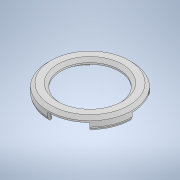
# Autodesk Inventor part: mirror_lock_v3
Saved by Autodesk Inventor 2020 (Build 240168000, 168)
## iProperties
Created: 2024-03-24
Part Number: mirror_lock_v3
Material: Типовые
Document SubType Name: Modeling
Designer: 4s
Density: 1 g/cm^3
Appearance: По умолчанию
Author: 4s
Autodesk Inventor part; units mm, degrees
ref_plane "YZ Plane" through (0, 0, 0) normal (1, 0, 0) x (0, 1, 0)
ref_plane "XZ Plane" through (0, 0, 0) normal (0, 1, 0) x (-1, 0, 0)
ref_plane "XY Plane" through (0, 0, 0) normal (0, 0, 1) x (1, 0, 0)
sketch "Эскиз1" plane through (0, 0, 0) normal (1, 0, 0) x (0, 1, 0)
  line L0 (0, 0) -> (10.522, 0) construction
  line L1 (0, 0) -> (0, -19) construction
  line L2 (0, 0) -> (0, -27.3) construction
  line L3 (0, -19) -> (3, -19)
  line L4 (3, -19) -> (3, -27.3)
  line L5 (3, -27.3) -> (0, -27.3)
  line L6 (0, -27.3) -> (0, -19)
  dimension "d0" = 19
  dimension "d1" = 27.3
  dimension "d2" = 3
  constraints: 14 end point, 2 horizontal, 2 parallel, 2 point on line, 1 perpendicular, 1 vertical
  measures "d0" distance of L0.start L1.end
  measures "d1" distance of L0.start L2.end
  measures "d2" distance of L4.end L5.end
revolve "Вращение1" add sketch "Эскиз1" angle 360 about axis through (0, 0, 0) along (0, 1, 0)
chamfer "Фаска1" distance 2 angle 45 1 edges at (0, 3, 19) measured on face at (2.1778, 3, -24.2689)
chamfer "Фаска2" distance 2 angle 45 1 edges at (0, 3, 27.3) measured on face at (3.853, 3, -24.7322)
sketch "Эскиз2" plane through (0, 0, 0) normal (1, 0, 0) x (0, 1, 0)
  line L0 (0, 0) -> (7.8289, 0) construction
  line L1 (0, 0) -> (0, -24.8) construction
  line L2 (0, 27.3) -> (0, -27.3) construction
  line L3 (0, -25.3) -> (-2.8173, -25.3)
  line L4 (0, -27.3) -> (-2.5558, -27.3)
  line L5 (-3.0173, -25.3) -> (-3.0173, -26.7) construction
  line L6 (0, -25.3) -> (0, -27.3)
  line L7 (-4.0346, 0.25) -> (-4.0346, -25) construction
  line L8 (-4.0346, -25) -> (-6, -25) construction
  arc A0 (-3.2173, -25.1) -> (-4.4555, -26.5989) centre (-4.0173, -25.7) ccw
  line L9 (-5.0173, -25) -> (-5.0173, 0) construction
  line L10 (-4.0346, -24.7) -> (-5.0173, -24.7) construction
  line L11 (-3.0173, -25.3) -> (-3.1008, -25.3) construction
  arc A1 (-3.0173, -25.7) -> (-3.1008, -25.3) centre (-4.0173, -25.7) ccw construction
  arc A2 (-3.2173, -25.1) -> (-2.8173, -25.3) centre (-2.8173, -24.8) ccw
  line L12 (-3.4322, -27.0978) -> (-4.4555, -26.5989)
  arc A3 (-4.4555, -26.5989) -> (-3.0173, -25.7) centre (-4.0173, -25.7) ccw construction
  arc A4 (-3.4322, -27.0978) -> (-2.5558, -27.3) centre (-2.5558, -25.3) ccw
  point P0 (-3.3032, -25)
  point P1 (-3.0173, -27.3)
  dimension "d10" = 24.8
  dimension "d11" = 3.017
  dimension "d12" = 0.5
  dimension "d14" = 4.035
  dimension "d15" = 2
  dimension "d16" = 0.983
  dimension "d17" = 0.3
  dimension "d18" = 0.5
  dimension "d19" = 50
  dimension "d21" = 3.017
  dimension "d22" = 2
  constraints: 24 end point, 13 point on circle, 10 point on line, 10 tangent, 6 horizontal, 5 centre point, 3 vertical, 1 collinear, 1 midpoint
  measures "d10" distance of L0.start L1.end
  measures "d12" distance from line of L1.end L3
  measures "d15" diameter of A0
  measures "d17" distance from line of point (-3.303, -25) L10
  measures "d18" radius of A2
  measures "d19" diameter of L8 L0
  measures "d22" radius of A4
revolve "Вращение2" add sketch "Эскиз2" angle 45 about axis through (0, 0, 0) along (0, -1, 0)
pattern_circular "Круговой массив1" count 4 over 360 about axis through (0, 1.5, 0) along (0, -1, 0) of "Вращение2"
